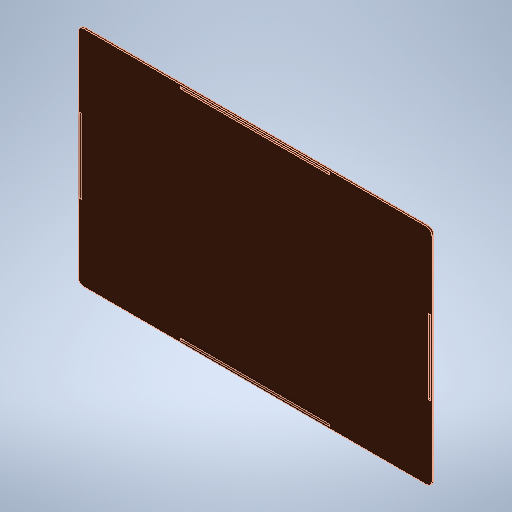
# Autodesk Inventor part: Base Full Game
Saved by Autodesk Inventor 2025.4 (Build 294407000, 407)
## iProperties
Created: 2026-05-09
Part Number: Base Full Game
Material: Generic
Document SubType Name: Sheet Metal
Designer: lenovo
Density: 1 g/cm^3
Sheet Metal Rule: Default_mm
Appearance: Default(1)
Author: lenovo
Autodesk Inventor part; units mm, degrees
ref_plane "YZ Plane" through (0, 0, 0) normal (1, 0, 0) x (0, 1, 0)
ref_plane "XZ Plane" through (0, 0, 0) normal (0, 1, 0) x (-1, 0, 0)
ref_plane "XY Plane" through (0, 0, 0) normal (0, 0, 1) x (1, 0, 0)
sketch "Sketch1" plane through (0, 0, 0) normal (0, 0, 1) x (1, 0, 0)
  line L0 (-475, -300) -> (475, -300)
  line L1 (475, -300) -> (475, 300)
  line L2 (475, 300) -> (-475, 300)
  line L3 (-475, 300) -> (-475, -300)
  line L4 (-475, -300) -> (475, 300) construction
  line L5 (475, -300) -> (-475, 300) construction
  point P0 (0, 0)
  dimension "d0" = 950
  dimension "d1" = 600
  measures "d0" distance of L2.end L1.end
  measures "d1" distance of L1.end L0.end
extrude "Plate1" add sketch "Sketch1" along normal blind 5
fillet "Corner Round1" radius 15 4 edges at (475, 300, 2.5) (475, -300, 2.5) (-475, -300, 2.5) (-475, 300, 2.5)
sketch "Sketch2" plane through (0, 0, 5) normal (0, 0, 1) x (1, 0, 0)
  line L0 (-475, 300) -> (-475, -300)
  line L1 (-475, 0) -> (475, 0)
  line L2 (475, -300) -> (475, 300)
  line L3 (475, 300) -> (-475, 300)
  line L4 (0, 300) -> (0, -300)
  line L5 (475, -300) -> (-475, -300)
  line L6 (-200, 295) -> (200, 295)
  line L7 (200, 295) -> (200, 289.92)
  line L8 (200, 289.92) -> (-200, 289.92)
  line L9 (-200, 289.92) -> (-200, 295)
  line L10 (-200, 295) -> (200, 289.92) construction
  line L11 (200, 295) -> (-200, 289.92) construction
  line L12 (-475, 300) -> (475, 300)
  line L13 (-470, -100) -> (-464.92, -100)
  line L14 (-464.92, -100) -> (-464.92, 100)
  line L15 (-464.92, 100) -> (-470, 100)
  line L16 (-470, 100) -> (-470, -100)
  line L17 (-470, -100) -> (-464.92, 100) construction
  line L18 (-464.92, -100) -> (-470, 100) construction
  line L19 (-475, -300) -> (-475, 300)
  line L20 (-200, -289.92) -> (-200, -295)
  line L21 (-200, -295) -> (200, -295)
  line L22 (200, -295) -> (200, -289.92)
  line L23 (-200, -295) -> (200, -289.92) construction
  line L24 (200, -295) -> (-200, -289.92) construction
  line L25 (200, -289.92) -> (-200, -289.92)
  line L26 (464.92, 100) -> (470, 100)
  line L27 (464.92, -100) -> (464.92, 100)
  line L28 (470, -100) -> (464.92, 100) construction
  line L29 (470, -100) -> (464.92, -100)
  line L30 (464.92, -100) -> (470, 100) construction
  line L31 (470, 100) -> (470, -100)
  point P0 (0, 0)
  point P1 (44.3571, 22.9179)
  point P2 (0, 292.46)
  point P3 (0, 295)
  point P4 (-467.46, 0)
  point P5 (-470, 0)
  point P6 (0, -292.46)
  point P7 (0, -295)
  point P8 (0, -300)
  point P9 (0, -300)
  point P10 (467.46, 0)
  point P11 (470, 0)
  point P12 (0, 0)
  dimension "d4" = 5.08
  dimension "d5" = 400
  dimension "d6" = 5
  dimension "d7" = 5.08
  dimension "d8" = 200
  dimension "d9" = 5
  dimension "d10" = 950
  dimension "d11" = 600
  constraints: 64 end point, 16 symmetric about line, 13 midpoint, 4 horizontal, 4 parallel, 3 vertical, 2 perpendicular, 2 point on line, 1 coincident
  measures "d4" distance between parallel lines of L6 L8
  measures "d5" distance of L6.start L7.start
  measures "d6" distance of point (0, 300) point (0, 295)
  measures "d7" distance of L15.end L15.start
  measures "d8" distance of L15.start L14.start
  measures "d9" distance of point (-475, 0) point (-470, 0)
  measures "d10" distance of L2.end L3.end
  measures "d11" distance of L2.start L2.end
extrude "Cut1" cut sketch "Sketch2" against normal blind 5 contours L16 L15 L14 L1 | L1 L14 L13 L16 | L6 L7 L8 L4 | L4 L8 L9 L6 | L21 L20 L25 L4 | L4 L25 L22 L21 | L31 L29 L27 L1 | L1 L27 L26 L31
equation "\"d14\" = Thickness"
equation "\"d2\" = Thickness"
equation "\"BendRadius\" = Thickness"
equation "\"BendReliefWidth\" = Thickness"
equation "\"BendReliefDepth\" = 0.5 * Thickness"
equation "\"TransitionRadius\" = BendRadius"
equation "\"JacobiRadiusSize\" = BendRadius"
equation "\"GapSize\" = Thickness"
equation "\"Thickness\" = 5"
body "Solid1"
